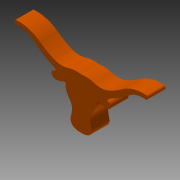
# Autodesk Inventor part: UT Longhorn
Saved by Autodesk Inventor 2014 (Build 180170000, 170)
## iProperties
Created: 2014-07-17
Part Number: UT Longhorn
Material: Generic
Document SubType Name: Modeling
Designer: quinn
Density: 1 g/cm^3
Appearance: Default
Author: quinn
Autodesk Inventor part; units mm, degrees
ref_plane "YZ Plane" through (0, 0, 0) normal (1, 0, 0) x (0, 1, 0)
ref_plane "Work Plane3" through (0, 0, 0) normal (0, 0, 1) x (1, 0, 0)
ref_plane "Work Plane1" through (0, 0, 0) normal (0, 0, 1) x (1, 0, 0)
sketch "Sketch3" plane through (0, 0, 0) normal (0, 0, 1) x (1, 0, 0)
  arc A0 (-14.4828, 15.2021) -> (-23.2609, 17.8276) centre (-22.2113, 5.3497) ccw
  arc A1 (-14.4828, 15.2021) -> (-9.7818, 12.5173) centre (-0.6814, 33.91) ccw
  arc A2 (0, 12.6617) -> (-4.532, 12.3207) centre (-1.5558, 3.0513) ccw
  arc A3 (-9.7818, 12.5173) -> (-4.532, 12.3207) centre (-6.8995, 19.293) ccw
  arc A4 (-23.2609, 17.8276) -> (-23.2609, 16.421) centre (-23.1237, 17.1243) ccw
  arc A5 (-19.2931, 15.9505) -> (-23.2609, 16.421) centre (-22.571, 5.2745) ccw
  arc A6 (-16.1338, 13.9003) -> (-19.2931, 15.9505) centre (-24.3961, 4.6276) ccw
  arc A7 (-16.1338, 13.9003) -> (-9.5198, 9.9718) centre (2.009, 36.9141) ccw
  arc A8 (-8.2989, 6.637) -> (-6.5467, 7.1491) centre (-9.6614, 14.5534) ccw
  arc A9 (-5.5396, 5.738) -> (-4.238, 3.0669) centre (4.0894, 8.7772) ccw
  arc A10 (-3.2758, 0.0944) -> (-4.238, 3.0669) centre (-7.1872, 0.4702) ccw
  arc A11 (-3.7397, -2.3677) -> (-3.2758, 0.0944) centre (-13.788, 0.8002) ccw
  arc A12 (-3.7397, -2.3677) -> (-2.6908, -4.9267) centre (-1.5092, -2.9479) ccw
  arc A13 (-2.6908, -4.9267) -> (0, -5.4558) centre (-0.4727, -0.7526) ccw
  arc A14 (-9.1718, 9.3717) -> (-9.5198, 9.9718) centre (-9.6221, 9.5115) ccw
  arc A15 (-5.9194, 7.4043) -> (-6.5467, 7.1491) centre (-5.9684, 6.6262) ccw
  arc A16 (-5.5121, 6.6262) -> (-5.9194, 7.4043) centre (-5.9596, 6.8876) ccw
  arc A17 (-5.5121, 6.6262) -> (-5.5396, 5.738) centre (-4.257, 6.1428) ccw
  arc A18 (-9.5198, 9.1003) -> (-9.1718, 9.3717) centre (-9.6345, 9.6062) ccw
  arc A19 (-9.5198, 9.1003) -> (-10.5011, 8.2893) centre (-9.1892, 7.7011) ccw
  arc A20 (-10.46, 7.3484) -> (-8.2989, 6.637) centre (-8.9924, 8.1686) ccw
  arc A21 (-10.5011, 8.2893) -> (-10.46, 7.3484) centre (-9.1849, 7.8754) ccw
  arc A22 (23.2609, 17.8276) -> (14.4829, 15.2021) centre (22.2114, 5.3497) ccw
  arc A23 (9.7819, 12.5173) -> (14.4829, 15.2021) centre (0.6815, 33.91) ccw
  arc A24 (4.5321, 12.3207) -> (0, 12.6617) centre (1.5558, 3.0513) ccw
  arc A25 (4.5321, 12.3207) -> (9.7819, 12.5173) centre (6.8996, 19.293) ccw
  arc A26 (23.2609, 16.421) -> (23.2609, 17.8276) centre (23.1237, 17.1243) ccw
  arc A27 (23.2609, 16.421) -> (19.2932, 15.9505) centre (22.5711, 5.2745) ccw
  arc A28 (19.2932, 15.9505) -> (16.1339, 13.9003) centre (24.3962, 4.6276) ccw
  arc A29 (9.5198, 9.9718) -> (16.1339, 13.9003) centre (-2.009, 36.9141) ccw
  arc A30 (6.5468, 7.1491) -> (8.299, 6.637) centre (9.6615, 14.5534) ccw
  arc A31 (4.2381, 3.0669) -> (5.5397, 5.738) centre (-4.0893, 8.7772) ccw
  arc A32 (4.2381, 3.0669) -> (3.2759, 0.0944) centre (7.1872, 0.4702) ccw
  arc A33 (3.2759, 0.0944) -> (3.7398, -2.3677) centre (13.788, 0.8002) ccw
  arc A34 (2.6908, -4.9267) -> (3.7398, -2.3677) centre (1.5093, -2.9479) ccw
  arc A35 (0, -5.4558) -> (2.6908, -4.9267) centre (0.4728, -0.7526) ccw
  arc A36 (9.5198, 9.9718) -> (9.1719, 9.3717) centre (9.6221, 9.5115) ccw
  arc A37 (6.5468, 7.1491) -> (5.9195, 7.4043) centre (5.9685, 6.6262) ccw
  arc A38 (5.9195, 7.4043) -> (5.5122, 6.6262) centre (5.9597, 6.8876) ccw
  arc A39 (5.5397, 5.738) -> (5.5122, 6.6262) centre (4.2571, 6.1428) ccw
  arc A40 (9.1719, 9.3717) -> (9.5198, 9.1003) centre (9.6346, 9.6062) ccw
  arc A41 (10.5012, 8.2893) -> (9.5198, 9.1003) centre (9.1893, 7.7011) ccw
  arc A42 (8.299, 6.637) -> (10.4601, 7.3484) centre (8.9925, 8.1686) ccw
  arc A43 (10.4601, 7.3484) -> (10.5012, 8.2893) centre (9.1849, 7.8754) ccw
  point P0 (0, 0)
  constraints: 88 point on circle, 44 centre point, 2 tangent
extrude "Extrusion2" add sketch "Sketch3" along normal blind 6.35
body "Solid2"
